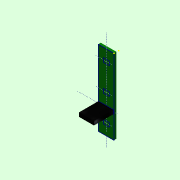
# Autodesk Inventor part: Sensor_Board_dummy
Saved by Autodesk Inventor 2015 (Build 190159000, 159)
## iProperties
Created: 2014-12-25
Part Number: Sensor_Board_dummy
Material: Generic
Document SubType Name: Modeling
Designer: Openlab
Density: 1 g/cm^3
Appearance: Dark Green
Mass: 2.2704 g
Surface Area: 29.3619 cm^2
Volume: 2.2704 cm^3
Author: Openlab
Autodesk Inventor part; units mm, degrees
ref_plane "YZ Plane" through (0, 0, 0) normal (1, 0, 0) x (0, 1, 0)
ref_plane "XZ Plane" through (0, 0, 0) normal (0, 1, 0) x (-1, 0, 0)
ref_plane "XY Plane" through (0, 0, 0) normal (0, 0, 1) x (1, 0, 0)
sketch "Sketch2" plane through (0, 0, 0) normal (0, 1, 0) x (-1, 0, 0)
  line L0 (10, 0) -> (0, 0)
  line L1 (0, 0) -> (0, -48)
  line L2 (0, -48) -> (10, -48)
  line L3 (10, -48) -> (10, 0)
  line L4 (6.9, -8.3) -> (3.1, -8.3)
  line L5 (3.1, -8.3) -> (3.1, -5.7)
  line L6 (3.1, -5.7) -> (6.9, -5.7)
  line L7 (6.9, -5.7) -> (6.9, -8.3)
  line L8 (6.9, -39.7) -> (3.1, -39.7)
  line L9 (3.1, -39.7) -> (3.1, -42.3)
  line L10 (3.1, -42.3) -> (6.9, -42.3)
  line L11 (6.9, -42.3) -> (6.9, -39.7)
  line L12 (3.1, -22.7) -> (6.9, -22.7)
  line L13 (3.1, -25.3) -> (3.1, -22.7)
  line L14 (6.9, -25.3) -> (3.1, -25.3)
  line L15 (6.9, -22.7) -> (6.9, -25.3)
  line L16 (23.6892, -32.5) -> (-2.3247, -32.5) construction
  line L17 (5, -54.7987) -> (5, -48.1542) construction
  line L18 (5, 9.3713) -> (5, -46.1174) construction
  line L19 (11.7769, -7) -> (1.25, -7) construction
  line L20 (11.7769, -24) -> (1.25, -24) construction
  line L21 (11.7769, -41) -> (1.25, -41) construction
  line L22 (9.75, -31.25) -> (0.25, -31.25)
  line L23 (0.25, -33.75) -> (9.75, -33.75)
  line L24 (9.75, -31.25) -> (9.75, -33.75)
  line L25 (0.25, -31.25) -> (0.25, -33.75)
  dimension "d0" = 10
  dimension "d1" = 48
  dimension "d13" = 3.8
  dimension "d14" = 2.6
  dimension "d40" = 5
  dimension "d49" = 15.5
  dimension "d50" = 7
  dimension "d51" = 24
  dimension "d52" = 41
  dimension "d53" = 2.5
  dimension "d54" = 9.5
  constraints: 52 end point, 9 horizontal, 8 parallel, 7 perpendicular, 4 equal length, 2 collinear, 2 vertical, 1 coincident, 8 other
  measures "d0" distance of L2.end L1.end
  measures "d1" distance of L1.end L0.end
  measures "d13" distance of L10.start L10.end
  measures "d14" distance of L9.start L10.start
  measures "d40" distance between parallel lines of L3 L17
  measures "d49" distance between parallel lines of L2 L16
  measures "d50" distance between parallel lines of L2 L21
  measures "d51" distance between parallel lines of L2 L20
  measures "d52" distance between parallel lines of L2 L19
  measures "d53" distance between parallel lines of L23 L22
  measures "d54" distance between parallel lines of L25 L24
extrude "Extrusion1" add sketch "Sketch2" along normal blind 1.6 contours L3 L2 L1 L0 | L4 L5 L6 L7 | L11 L10 L9 L8 | L12 L15 L14 L13 | L24 L23 L25 L22
extrude "Extrusion4" add sketch "Sketch2" along normal blind 2.98 contours L4 L5 L6 L7 | L11 L10 L9 L8 | L12 L15 L14 L13
sketch "Sketch3" plane through (0, 2.98, 0) normal (0, 1, 0) x (1, 0, 0)
  line L0 (-3.1, 25.3) -> (-6.9, 25.3) construction
  line L1 (-6.9, 22.7) -> (-3.1, 22.7) construction
  point P0 (0, 0)
  point P1 (-5.1459, 24.0493)
extrude "Extrusion5" add sketch "Sketch2" against normal blind 12.5 contours L24 L23 L25 L22
body "Solid1"
